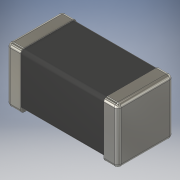
# Autodesk Inventor part: Resistor_1608-0.5mm
Saved by Autodesk Inventor 2018 (Build 220112000, 112)
## iProperties
Created: 2016-08-15
Part Number: Resistor_1608-0.5mm
Material: Copper
Document SubType Name: Modeling
Designer: Bradley
Density: 8.94 g/cm^3
Appearance: Smooth - Black
Author: Bradley
Autodesk Inventor part; units mm, degrees
ref_plane "YZ Plane" through (0, 0, 0) normal (1, 0, 0) x (0, 1, 0)
ref_plane "XZ Plane" through (0, 0, 0) normal (0, 1, 0) x (-1, 0, 0)
ref_plane "XY Plane" through (0, 0, 0) normal (0, 0, 1) x (1, 0, 0)
sketch "Sketch1" plane through (0, 0, 0) normal (0, 0, 1) x (1, 0, 0)
  line L0 (-0.8, 0.75) -> (-0.6, 0.75)
  line L1 (-0.6, 0.75) -> (-0.6, -0.05)
  line L2 (-0.6, -0.05) -> (-0.8, -0.05)
  line L3 (-0.8, -0.05) -> (-0.8, 0.75)
  line L4 (-0.6, 0.74) -> (0.6, 0.74)
  line L5 (0.6, 0.74) -> (0.6, 0)
  line L6 (0.6, 0) -> (-0.6, 0)
  line L7 (-0.6, 0) -> (-0.6, 0.74)
  line L8 (0.6, 0.75) -> (0.8, 0.75)
  line L9 (0.8, 0.75) -> (0.8, -0.05)
  line L10 (0.8, -0.05) -> (0.6, -0.05)
  line L11 (0.6, -0.05) -> (0.6, 0.75)
  point P0 (0, 0)
  point P1 (0, 0.74)
  point P2 (0, 0)
  dimension "d0" = 1.6
  dimension "d1" = 0.8
  dimension "d2" = 0.2
  dimension "d3" = 0.05
  dimension "d6" = 0.01
  constraints: 24 end point, 6 parallel, 3 horizontal, 3 perpendicular, 3 point on line, 2 collinear, 2 midpoint, 1 coincident, 1 vertical alignment
  measures "d0" distance between parallel lines of L9 L3
  measures "d1" distance of L2.end L0.start
  measures "d2" distance of L1.end L2.end
  measures "d3" distance between parallel lines of L2 L6
  measures "d6" distance between parallel lines of L4 L0
extrude "Extrusion1" add sketch "Sketch1" along normal mid plane 0.8 contours L0 L1 L2 L3 | L11 L8 L9 L10 L5
extrude "Extrusion2" add sketch "Sketch1" along normal mid plane 0.79 contours L4 L5 L6 L1
fillet "Fillet2" radius 0.05 4 edges at (0, 0.74, 0.395) (0, 0, 0.395) (0, 0.74, -0.395) (0, 0, -0.395)
fillet "Fillet1" radius 0.05 16 edges at (-0.7, 0.75, 0.4) (0.7, 0.75, 0.4) (-0.7, 0.75, -0.4) (0.7, 0.75, -0.4) (0.8, 0.75, 0) (0.8, 0.35, -0.4) (0.8, -0.05, 0) (0.7, -0.05, -0.4) (0.7, -0.05, 0.4) (0.8, 0.35, 0.4) (-0.7, -0.05, -0.4) (-0.8, -0.05, 0) (-0.8, 0.35, 0.4) (-0.7, -0.05, 0.4) (-0.8, 0.35, -0.4) (-0.8, 0.75, 0)
body "Solid1"
